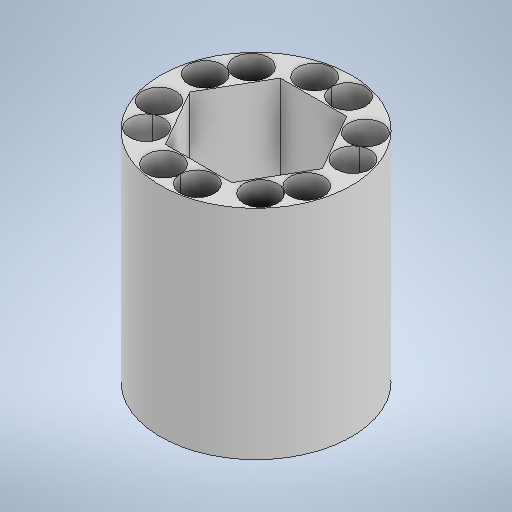
# Autodesk Inventor part: alumina caseing
Saved by Autodesk Inventor 2025.2 (Build 292293000, 293)
## iProperties
Created: 2025-04-27
Part Number: alumina caseing
Material: Generic
Document SubType Name: Modeling
Designer: alex
Density: 1 g/cm^3
Appearance: Default
Author: alex
Autodesk Inventor part; units mm, degrees
ref_plane "YZ Plane" through (0, 0, 0) normal (1, 0, 0) x (0, 1, 0)
ref_plane "XZ Plane" through (0, 0, 0) normal (0, 1, 0) x (-1, 0, 0)
ref_plane "XY Plane" through (0, 0, 0) normal (0, 0, 1) x (1, 0, 0)
sketch "Sketch1" plane through (0, 0, 0) normal (0, 1, 0) x (-1, 0, 0)
  line L0 (-560.0298, 0) -> (-280.0149, 485)
  line L1 (-280.0149, 485) -> (280.0149, 485)
  line L2 (280.0149, 485) -> (560.0298, 0)
  line L3 (560.0298, 0) -> (280.0149, -485)
  line L4 (280.0149, -485) -> (-280.0149, -485)
  line L5 (-280.0149, -485) -> (-560.0298, 0)
  line L6 (0, 485) -> (280.0149, 485)
  line L7 (0, 485) -> (-280.0149, 485)
  line L8 (-280.0149, 485) -> (-420.0223, 242.5)
  line L9 (-420.0223, 242.5) -> (-560.0298, 0)
  line L10 (-560.0298, 0) -> (-420.0223, -242.5)
  line L11 (-420.0223, -242.5) -> (-280.0149, -485)
  line L12 (-280.0149, -485) -> (0, -485)
  line L13 (0, -485) -> (280.0149, -485)
  line L14 (280.0149, -485) -> (420.0223, -242.5)
  line L15 (420.0223, -242.5) -> (560.0298, 0)
  line L16 (560.0298, 0) -> (420.0223, 242.5)
  line L17 (420.0223, 242.5) -> (280.0149, 485)
  circle A0 centre (140.0074, 625.0074) radius 140.0074
  circle A1 centre (-140.0074, 625.0074) radius 140.0074
  circle A2 centre (-471.2686, 433.7537) radius 140.0074
  circle A3 centre (-611.276, 191.2537) radius 140.0074
  line L18 (-560.0298, 0) -> (-639.9785, 0)
  circle A4 centre (471.2686, 433.7537) radius 140.0074
  circle A5 centre (611.276, 191.2537) radius 140.0074
  line L19 (280.0149, 485) -> (613.8502, 677.7399)
  line L20 (-280.0149, 485) -> (-280.0149, 1036.6833)
  line L21 (-560.0298, 0) -> (-952.9053, 226.8268)
  line L22 (-280.0149, 485) -> (-615.2161, 678.5285)
  line L23 (280.0149, 485) -> (280.0149, 1486.2833)
  line L24 (560.0298, 0) -> (896.7053, 194.3797)
  circle A6 centre (140.0074, -625.0074) radius 140.0074
  circle A7 centre (-140.0074, -625.0074) radius 140.0074
  circle A8 centre (-471.2686, -433.7537) radius 140.0074
  circle A9 centre (-611.276, -191.2537) radius 140.0074
  circle A10 centre (471.2686, -433.7537) radius 140.0074
  circle A11 centre (611.276, -191.2537) radius 140.0074
  circle A12 centre (0, 0) radius 790
  line L25 (-548.4828, 0) -> (-274.2414, 475)
  line L26 (-274.2414, 475) -> (274.2414, 475)
  line L27 (274.2414, 475) -> (548.4828, 0)
  line L28 (548.4828, 0) -> (274.2414, -475)
  line L29 (274.2414, -475) -> (-274.2414, -475)
  line L30 (-274.2414, -475) -> (-548.4828, 0)
  line L31 (-539.5916, 0) -> (-269.7958, 467.3)
  line L32 (-269.7958, 467.3) -> (269.7958, 467.3)
  line L33 (269.7958, 467.3) -> (539.5916, 0)
  line L34 (539.5916, 0) -> (269.7958, -467.3)
  line L35 (269.7958, -467.3) -> (-269.7958, -467.3)
  line L36 (-269.7958, -467.3) -> (-539.5916, 0)
  point P0 (0, 625.0074)
  point P1 (140.0074, 485)
  point P2 (350.0186, 363.75)
  point P3 (541.2723, 312.5037)
  point P4 (490.026, 121.25)
  point P5 (490.026, -121.25)
  point P6 (541.2723, -312.5037)
  point P7 (350.0186, -363.75)
  point P8 (140.0074, -485)
  point P9 (0, -625.0074)
  point P10 (-140.0074, -485)
  point P11 (-350.0186, -363.75)
  point P12 (-541.2723, -312.5037)
  point P13 (-490.026, -121.25)
  point P14 (-490.026, 121.25)
  point P15 (-541.2723, 312.5037)
  point P16 (-350.0186, 363.75)
  point P17 (-140.0074, 485)
  dimension "d0" = 485
  dimension "d13" = 90
  dimension "d14" = 90
  dimension "d15" = 90
  dimension "d24" = 475
  dimension "d26" = 467.3
  dimension "d27" = 1580
  constraints: 74 end point, 15 tangent, 13 centre point, 6 collinear, 6 midpoint, 6 symmetric about line, 4 coincident, 3 equal radius, 3 horizontal, 1 perpendicular, 1 vertical, 45 other
  measures "d0" distance from line of L1 point (0, 0)
  measures "d13" angle of L19 L2
  measures "d14" angle of L0 L21
  measures "d15" angle of L8 L22
  measures "d24" distance from line of point (0, 0) L26
  measures "d26" distance from line of L32 point (0, 0)
  measures "d27" diameter of A12
extrude "Extrusion1" add sketch "Sketch1" along normal blind 1800 contours L21 A3 L0 | L0 L1 L2 L3 L4 L5 | L5 A9 A8 L4 A7 A6 L3 A10 A11 L24 A12 L21 | A3 A2 L0 | L5 A8 A9 | L21 A12 L22 A2 A3 | A2 L22 L0 | L22 A12 L20 | L20 A1 L1 | A12 L23 A0 A1 L20 | L24 A5 A4 L19 A12 | A1 A0 L1 | L4 A6 A7 | A12 L19 L23 | L24 L2 A5 | L23 L1 A0 | L2 A4 A5 | A4 L2 L19 | A11 A10 L3
body "Solid1"
